weihnachtshaken (Autodesk Fusion 360 design; units mm, degrees)
Autodesk Fusion 360 part; units mm, degrees
sketch "Sketch1" plane through (0, 0, 0) normal (0, 0, 1) x (1, 0, 0)
  line L0 (0, 0) -> (21, 0)
  line L1 (21, 0) -> (21, 2)
  line L2 (21, 2) -> (0, 2)
  line L3 (0, 2) -> (0, 0)
  line L4 (0, 2) -> (2, 2)
  line L5 (2, 2) -> (2, -18)
  line L6 (2, -18) -> (0, -18)
  line L7 (0, -18) -> (0, 2)
  line L8 (21, 2) -> (19, 2)
  line L9 (19, 2) -> (19, -23)
  line L10 (19, -23) -> (21, -23)
  line L11 (21, -23) -> (21, 2)
  line L12 (19, -23) -> (34, -23)
  line L13 (34, -23) -> (34, -25)
  line L14 (34, -25) -> (19, -25)
  line L15 (19, -25) -> (19, -23)
  line L16 (34, -23) -> (32, -23)
  line L17 (32, -23) -> (32, -11)
  line L18 (32, -11) -> (34, -11)
  line L19 (34, -11) -> (34, -23)
  dimension "d1" = 21
  dimension "d2" = 2
  dimension "d3" = 2
  dimension "d4" = 20
  dimension "d5" = 2
  dimension "d6" = 25
  dimension "d7" = 15
  dimension "d8" = 2
  dimension "d9" = 2
  dimension "d10" = 12
  constraint horizontal L0
  constraint vertical L1
  constraint horizontal L2
  constraint vertical L3
  constraint coincident L0.start L3.end
  constraint horizontal L4
  constraint vertical L5
  constraint horizontal L6
  constraint vertical L7
  constraint horizontal L8
  constraint vertical L9
  constraint horizontal L10
  constraint vertical L11
  constraint horizontal L12
  constraint vertical L13
  constraint horizontal L14
  constraint vertical L15
  constraint horizontal L16
  constraint vertical L17
  constraint horizontal L18
  constraint vertical L19
  measures "d1" distance of L0.start L0.end
  measures "d2" distance of L0.start L2.end
  measures "d3" distance of L2.end L4.end
  measures "d4" distance of L2.end L6.end
  measures "d5" distance of L1.end L8.end
  measures "d6" distance of L1.end L10.end
  measures "d7" distance of L9.end L12.end
  measures "d8" distance of L9.end L14.end
  measures "d9" distance of L12.end L16.end
  measures "d10" distance of L12.end L18.end
extrude "Extrude1" add sketch "Sketch1" along normal blind 10
fillet "Fillet1" radius 4 2 edges at (21, -23, 5) (32, -23, 5)
